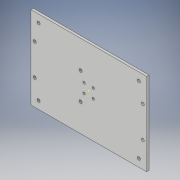
# Autodesk Inventor part: Plancha Inferior
Saved by Autodesk Inventor 2019 (Build 230136000, 136)
## iProperties
Created: 2019-05-15
Part Number: Plancha Inferior
Material: Generic
Document SubType Name: Modeling
Designer: Iván
Density: 1 g/cm^3
Appearance: Default
Author: Iván
Autodesk Inventor part; units mm, degrees
ref_plane "YZ Plane" through (0, 0, 0) normal (1, 0, 0) x (0, 1, 0)
ref_plane "XZ Plane" through (0, 0, 0) normal (0, 1, 0) x (-1, 0, 0)
ref_plane "XY Plane" through (0, 0, 0) normal (0, 0, 1) x (1, 0, 0)
sketch "Sketch1" plane through (0, 0, 0) normal (0, 0, 1) x (1, 0, 0)
  line L0 (-75, 53.5) -> (75, 53.5)
  line L1 (75, 53.5) -> (75, -53.5)
  line L2 (75, -53.5) -> (-75, -53.5)
  line L3 (-75, -53.5) -> (-75, 53.5)
  point P0 (0, 0)
  point P1 (0, -53.5)
  point P2 (75, 0)
  dimension "d0" = 150
  dimension "d1" = 107
  constraints: 8 end point, 2 midpoint, 2 parallel, 1 horizontal, 1 horizontal alignment, 1 perpendicular, 1 vertical alignment
  measures "d0" distance of L0.start L0.end
  measures "d1" distance of L0.end L1.end
extrude "Extrusion1" add sketch "Sketch1" along normal blind 3.175
sketch "Sketch2" plane through (0, 0, 3.175) normal (0, 0, 1) x (1, 0, 0)
  circle A0 centre (-65, 43.5) radius 2
  line L0 (75, 53.5) -> (-75, 53.5) projected
  line L1 (-75, 53.5) -> (-75, -53.5) projected
  circle A1 centre (-65, -43.5) radius 2
  line L2 (-75, -53.5) -> (75, -53.5) projected
  circle A2 centre (-70, 20.25) radius 2
  circle A3 centre (-70, -20.25) radius 2
  circle A4 centre (-10.5, 17.5) radius 2
  circle A5 centre (-10.5, -17.5) radius 2
  circle A6 centre (-6, 6) radius 1.5
  circle A7 centre (-6, -6) radius 1.5
  circle A8 centre (6, 6) radius 1.5
  circle A9 centre (6, -6) radius 1.5
  line L3 (0, 53.5) -> (0, -53.5)
  circle A10 centre (65, 43.5) radius 2
  circle A11 centre (65, -43.5) radius 2
  circle A12 centre (70, 20.25) radius 2
  circle A13 centre (70, -20.25) radius 2
  point P0 (0, 0)
  dimension "d4" = 4
  dimension "d5" = 10
  dimension "d6" = 10
  dimension "d7" = 10
  dimension "d8" = 10
  dimension "d9" = 33.25
  dimension "d10" = 5
  dimension "d11" = 5
  dimension "d13" = 40.5
  dimension "d14" = 4
  dimension "d15" = 36
  dimension "d16" = 64.5
  dimension "d18" = 35
  dimension "d19" = 3
  dimension "d20" = 6
  dimension "d21" = 6
  dimension "d22" = 6
  dimension "d23" = 6
  constraints: 14 centre point, 7 equal radius, 4 symmetric about line, 3 vertical alignment, 2 end point, 2 horizontal alignment, 2 midpoint, 4 other
  measures "d4" diameter of A0
  measures "d5" distance from line of L0 A0.centre
  measures "d6" distance from line of A0.centre L1
  measures "d7" distance from line of L1 A1.centre
  measures "d8" distance from line of L2 A1.centre
  measures "d9" distance from line of L0 A2.centre
  measures "d10" distance from line of L1 A2.centre
  measures "d11" distance from line of L1 A3.centre
  measures "d13" distance of A3.centre A2.centre
  measures "d14" diameter of A4
  measures "d15" distance from line of L0 A4.centre
  measures "d16" distance from line of L1 A4.centre
  measures "d18" distance of A5.centre A4.centre
  measures "d19" diameter of A6
  measures "d20" horizontal distance of point (0, 0) A6.centre
  measures "d21" horizontal distance of point (0, 0) A6.centre
  measures "d22" horizontal distance of A7.centre point (0, 0)
  measures "d23" horizontal distance of point (0, 0) A8.centre
extrude "Extrusion2" cut sketch "Sketch2" against normal through all contours A0 | A1 | A2 | A3 | A4 | A5 | A6 | A7 | A8 | A9 | A10 | A11 | A12 | A13
sketch "Sketch3" plane through (0, 0, 3.175) normal (0, 0, 1) x (1, 0, 0)
  point P0 (0, 0)
equation "\"d7\" = d6"
equation "\"d8\" = d5"
equation "\"d11\" = d10"
equation "\"d14\" = d4"
equation "\"d21\" = d20"
equation "\"d22\" = d20"
equation "\"d23\" = d21"
body "Solid1"
